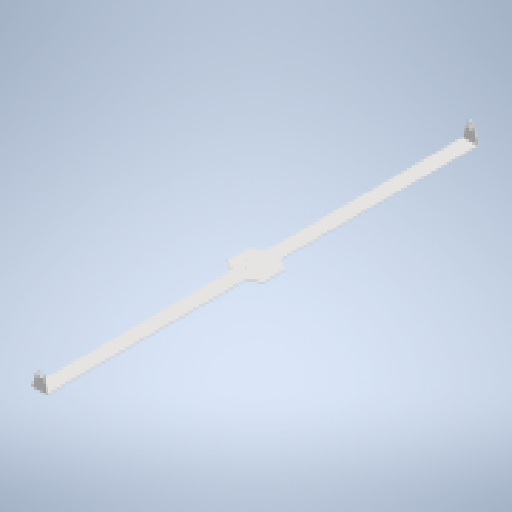
# Autodesk Inventor part: Suporte Central Atualizado
Saved by Autodesk Inventor 2024 (Build 280153000, 153)
## iProperties
Created: 2024-05-08
Part Number: Suporte Central Atualizado
Material: Genérico
Document SubType Name: Modeling
Designer: mathe
Density: 1 g/cm^3
Appearance: Padrão
Author: mathe
Autodesk Inventor part; units mm, degrees
ref_plane "YZ Plane" through (0, 0, 0) normal (1, 0, 0) x (0, 1, 0)
ref_plane "XZ Plane" through (0, 0, 0) normal (0, 1, 0) x (-1, 0, 0)
ref_plane "XY Plane" through (0, 0, 0) normal (0, 0, 1) x (1, 0, 0)
sketch "Esboço1" plane through (0, 0, 0) normal (0, 1, 0) x (-1, 0, 0)
  line L0 (-56.1514, 755.3759) -> (-111.1514, 755.3759)
  line L1 (-111.1514, 755.3759) -> (-111.1514, -847.6241)
  line L2 (-111.1514, -847.6241) -> (-56.1514, -847.6241)
  line L3 (-56.1514, -847.6241) -> (-56.1514, 755.3759)
  point P0 (0, 0)
  dimension "d0" = 1603
  dimension "d1" = 55
  constraints: 8 end point, 2 parallel, 1 horizontal, 1 perpendicular
  measures "d0" distance between parallel lines of L2 L0
  measures "d1" distance between parallel lines of L1 L3
extrude "Extrusão1" add sketch "Esboço1" along normal blind 3
sketch "Esboço2" plane through (56.1514, 0, 755.3759) normal (0, 0, 1) x (1, 0, 0)
  circle A0 centre (28.1143, 53) radius 12.5
  circle A1 centre (28.1143, 53) radius 11
  line L0 (55, 3) -> (0, 3) projected
  line L1 (0, 3) -> (15.6143, 53)
  line L2 (40.6143, 53) -> (55, 3)
  point P0 (-56.1514, 0)
  point P1 (17.1143, 53)
  point P2 (39.1143, 53)
  dimension "d4" = 25
  dimension "d5" = 22
  dimension "d8" = 50
  constraints: 4 end point, 4 point on circle, 2 centre point, 1 coincident
  measures "d4" diameter of A0
  measures "d5" diameter of A1
  measures "d8" distance from line of L0 A0.centre
extrude "Extrusão2" add sketch "Esboço2" against normal blind 3 contours L2 L0 L1 A0
sketch "Esboço4" plane through (111.1514, 0, -847.6241) normal (0, 0, -1) x (-1, 0, 0)
  arc A0 (39.3857, 53) -> (14.3857, 53) centre (26.8857, 53) ccw projected
  line L0 (0, 3) -> (55, 3)
  circle A1 centre (26.8857, 53) radius 11
  circle A2 centre (26.8857, 53) radius 12.5
  line L1 (14.3857, 53) -> (0, 3)
  line L2 (55, 3) -> (39.3857, 53)
  point P0 (111.1514, 0)
  dimension "d40" = 22
  constraints: 6 end point, 2 coincident, 1 centre point, 1 horizontal, 1 horizontal alignment, 3 other
  measures "d40" diameter of A1
extrude "Extrusão3" add sketch "Esboço4" against normal blind 3
sketch "Esboço5" plane through (0, 3, 0) normal (0, 1, 0) x (1, 0, 0)
  line L0 (56.1514, -749.3759) -> (95.2658, -749.3759) projected
  line L1 (111.1514, 844.6241) -> (56.1514, 844.6241) projected
  line L2 (56.1514, 847.6241) -> (56.1514, -755.3759) projected
  circle A0 centre (-124.6549, -214.6876) radius 2
  circle A1 centre (-96.9649, -152.5807) radius 2
  line L3 (16.1057, 85.4763) -> (84.2658, 124.8286)
  line L4 (84.2658, 124.8286) -> (152.4258, 85.4763)
  line L5 (152.4258, 85.4763) -> (152.4258, 6.7718)
  line L6 (152.4258, 6.7718) -> (84.2658, -32.5804)
  line L7 (84.2658, -32.5804) -> (16.1057, 6.7718)
  line L8 (16.1057, 6.7718) -> (16.1057, 85.4763)
  line L9 (56.1514, 847.6241) -> (56.1514, -755.3759) projected
  line L10 (111.1514, -755.3759) -> (111.1514, 847.6241) projected
  line L11 (56.1514, -755.3759) -> (111.1514, -755.3759)
  line L12 (111.1514, -755.3759) -> (111.1514, 847.6241)
  line L13 (111.1514, 847.6241) -> (56.1514, 847.6241)
  line L14 (56.1514, 847.6241) -> (56.1514, -755.3759)
  line L15 (95.2658, -755.3759) -> (95.2658, -755.3759) projected
  line L16 (90.2658, 847.6241) -> (78.2658, 847.6241) projected
  line L17 (95.2658, -752.3759) -> (95.2658, -752.3759) projected
  point P0 (111.1514, 841.6241)
  point P1 (56.1514, 841.6241)
  point P2 (84.2658, 46.1241)
  point P3 (73.2658, -755.3759)
  point P4 (73.2658, -755.3759)
  point P5 (84.2658, -755.3759)
  point P6 (84.2658, 847.6241)
  point P7 (84.2658, 847.6241)
  point P8 (73.2658, -752.3759)
  point P9 (84.2658, -752.3759)
  point P10 (111.1514, 109.3061)
  point P11 (111.1514, -17.058)
  point P12 (56.1514, -16.3486)
  point P13 (56.1514, 108.5967)
  dimension "d13" = 4
  dimension "d14" = 4
  dimension "d15" = 68
  dimension "d20" = 722.7955
  dimension "d22" = 722.7955
  dimension "d25" = 0
  constraints: 20 end point, 2 centre point, 2 midpoint, 2 parallel, 1 horizontal, 1 perpendicular, 18 other
  measures "d13" diameter of A1
  measures "d14" diameter of A0
  measures "d15" distance of A0.centre A1.centre
  measures "d20" distance of point (84.266, -755.376) L6.end
  measures "d22" distance of point (84.266, 847.624) L3.end
  measures "d25" horizontal distance of point (84.266, -752.376) point (84.266, 46.124)
extrude "Extrusão4" add sketch "Esboço5" against normal blind 3 contours L4 L5 L6 L10 | L2 L7 L8 L3
sketch "Esboço6" plane through (0, 3, 0) normal (0, 1, 0) x (1, 0, 0)
  circle A0 centre (116.2657, 46.1244) radius 1.5
  circle A1 centre (52.2657, 46.1244) radius 1.5
  line L0 (16.1057, 85.4763) -> (16.1057, 6.7718) projected
  line L1 (152.4258, 6.7718) -> (152.4258, 85.4763) projected
  circle A2 centre (81.9973, 14.1244) radius 1.5
  circle A3 centre (81.9973, 78.1244) radius 1.5
  point P0 (0, 0)
  point P1 (56.1514, -16.3486)
  point P2 (56.1514, 108.5967)
  dimension "d28" = 3
  dimension "d29" = 3
  dimension "d30" = 64
  dimension "d31" = 36.16
  dimension "d43" = 3
  dimension "d44" = 3
  dimension "d45" = 64
  dimension "d46" = 32
  dimension "d47" = 32
  dimension "d48" = 36.1602
  dimension "d49" = 62.473
  constraints: 4 centre point
  measures "d28" diameter of A1
  measures "d29" diameter of A0
  measures "d30" distance of A0.centre A1.centre
  measures "d31" distance from line of L0 A1.centre
  measures "d43" diameter of A2
  measures "d44" diameter of A3
  measures "d45" distance of A3.centre A2.centre
  measures "d46" vertical distance of A1.centre A2.centre
  measures "d47" vertical distance of A3.centre A1.centre
  measures "d48" distance from line of L1 A0.centre
  measures "d49" vertical distance of point (56.151, -16.349) A1.centre
hole "Furo1" at (52.2657, 3, -46.1244) at (116.2657, 3, -46.1244) at (81.9973, 3, -14.1244) at (81.9973, 3, -78.1244) direction (0, -1, 0) diameter 3 depth 20 tip angle 118
extrude "Extrusão5" add sketch "Esboço2" against normal blind 3 contours A0
